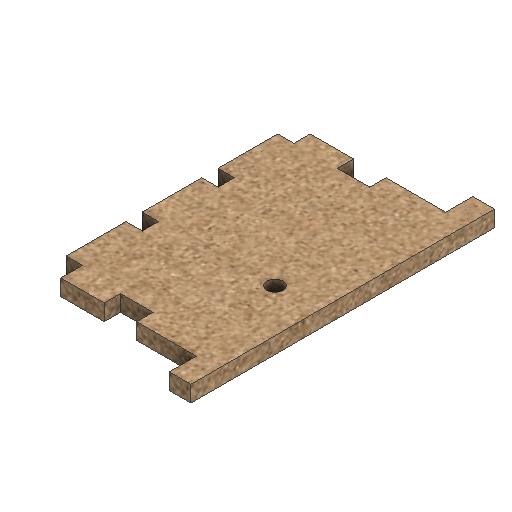
# Autodesk Inventor part: side_wall
Saved by Autodesk Inventor 2024 (Build 280153000, 153)
## iProperties
Created: 2024-06-06
Part Number: side_wall
Material: MDF Medium Density Fiberboard
Document SubType Name: Modeling
Designer: USER
Density: 0.8 g/cm^3
Appearance: Cardboard - Corrugated
Mass: 3.43184 g
Surface Area: 34.8814 cm^2
Volume: 4.28979 cm^3
Author: USER
Autodesk Inventor part; units mm, degrees
ref_plane "YZ Plane" through (0, 0, 0) normal (1, 0, 0) x (0, 1, 0)
ref_plane "XZ Plane" through (0, 0, 0) normal (0, 1, 0) x (-1, 0, 0)
ref_plane "XY Plane" through (0, 0, 0) normal (0, 0, 1) x (1, 0, 0)
sketch "草圖3" plane through (0, 0, 0) normal (0, 1, 0) x (-1, 0, 0)
  line L0 (0, 0) -> (25, 0)
  line L1 (25, 0) -> (25, -31)
  line L2 (25, -31) -> (0, -31)
  line L3 (0, -31) -> (0, 0)
  circle A0 centre (4, -3.5) radius 1.5
  line L4 (28, -3) -> (25, -3)
  line L5 (25, -3) -> (25, -28)
  line L6 (25, -28) -> (28, -28)
  line L7 (28, -28) -> (28, -3)
  line L8 (28, -14) -> (25, -14)
  line L9 (25, -14) -> (25, -17)
  line L10 (25, -17) -> (28, -17)
  line L11 (28, -17) -> (28, -14)
  line L12 (25, 0) -> (0, 0)
  line L13 (0, 0) -> (0, 15)
  line L14 (0, 15) -> (25, 15)
  line L15 (25, 15) -> (25, 0)
  line L16 (28, 11) -> (25, 11)
  line L17 (25, 11) -> (25, 0)
  line L18 (25, 0) -> (28, 0)
  line L19 (28, 0) -> (28, 11)
  line L20 (0, 15) -> (0, 20)
  line L21 (0, 20) -> (-4, 20)
  line L22 (-4, 20) -> (-4, -31)
  line L23 (-4, -31) -> (-4, -36)
  line L24 (-4, -36) -> (0, -36)
  line L25 (0, -36) -> (0, -31)
  line L26 (17, 15) -> (11, 15)
  line L27 (11, 15) -> (11, 12)
  line L28 (11, 12) -> (17, 12)
  line L29 (17, 12) -> (17, 15)
  line L30 (17, -28) -> (11, -28)
  line L31 (11, -28) -> (11, -31)
  line L32 (11, -31) -> (17, -31)
  line L33 (17, -31) -> (17, -28)
  point P0 (25, -15.5)
  point P1 (25, -15.5)
  point P2 (17, -31)
  dimension "d20" = 25
  dimension "d24" = 27.5
  dimension "d25" = 21
  dimension "d26" = 3
  dimension "d27" = 3
  dimension "d28" = 3
  dimension "d29" = 3
  dimension "d30" = 3
  dimension "d31" = 3
  dimension "d33" = 3
  dimension "d34" = 11
  dimension "d35" = 5
  dimension "d36" = 4
  dimension "d37" = 5
  dimension "d38" = 3
  dimension "d39" = 6
  dimension "d40" = 3
  dimension "d41" = 8
  constraints: 68 end point, 14 parallel, 11 perpendicular, 7 horizontal, 6 point on line, 4 midpoint, 1 centre point, 1 vertical
  measures "d20" distance of L1.end L2.end
  measures "d24" distance from line of L2 A0.centre
  measures "d25" distance from line of L1 A0.centre
  measures "d26" diameter of A0
  measures "d27" distance from line of L1.end L6
  measures "d28" distance of L0.end L4.end
  measures "d29" distance of L4.start L4.end
  measures "d30" distance of L9.end L10.end
  measures "d31" distance of L8.end L9.end
  measures "d33" distance of L0.end L18.end
  measures "d34" distance of L0.end L16.end
  measures "d35" distance of L13.end L20.end
  measures "d36" distance of L20.end L21.end
  measures "d37" distance of L22.end L23.end
  measures "d38" distance of L30.end L31.end
  measures "d39" distance of L31.end L32.end
  measures "d40" distance of L28.end L26.start
  measures "d41" distance between parallel lines of L15 L29
extrude "擠出4" add sketch "草圖3" along normal blind 3 contours L13 L14 L27 L28 L29 L15 L0 | L0 L1 L2 L33 L30 L31 L3 | L3 L25 L24 L23 L22 L21 L20 L13 | L15 L16 L19 L18 | L4 L7 L8 L1 | L10 L7 L6 L1
